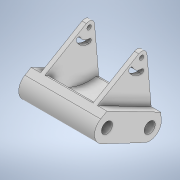
# Autodesk Inventor part: Kauri camera predator mini standoff mount
Saved by Autodesk Inventor 2020 (Build 240168000, 168)
## iProperties
Created: 2022-05-05
Part Number: Kauri camera predator mini standoff mount
Material: Generic
Document SubType Name: Modeling
Designer: Steven
Density: 1 g/cm^3
Appearance: Default
Author: Steven
Autodesk Inventor part; units mm, degrees
ref_plane "YZ Plane" through (0, 0, 0) normal (1, 0, 0) x (0, 1, 0)
ref_plane "XZ Plane" through (0, 0, 0) normal (0, 1, 0) x (-1, 0, 0)
ref_plane "XY Plane" through (0, 0, 0) normal (0, 0, 1) x (1, 0, 0)
sketch "Sketch1" plane through (0, 0, 0) normal (1, 0, 0) x (0, 1, 0)
  circle A0 centre (-9.7574, -19.7073) radius 1.55 construction
  circle A1 centre (0, 0) radius 1.55 construction
  circle A2 centre (-9.7574, -19.7073) radius 2.55
  circle A3 centre (0, 0) radius 2.55
  arc A4 (-12.2239, -24.4871) -> (-4.9776, -22.1738) centre (-9.7574, -19.7073) ccw
  circle A5 centre (0, 0) radius 5.7448
  line L0 (-4.9776, -22.1738) -> (5.1052, -2.6344)
  arc A6 (-4.9776, -22.1738) -> (-12.2239, -24.4871) centre (-9.7574, -19.7073) ccw
  line L1 (-14.5372, -17.2408) -> (-5.1904, 2.4623)
  line L2 (0, 0) -> (0, -35.9972) construction
  dimension "d0" = 5.1
  dimension "d1" = 5.1
  constraints: 7 centre point, 7 point on circle, 6 end point, 4 coincident, 1 tangent, 1 vertical
  measures "d0" diameter of A2
  measures "d1" diameter of A3
extrude "Extrusion1" add sketch "Sketch1" along normal blind 35
sketch "Sketch2" plane through (35, 0, 0) normal (1, 0, 0) x (0, 0, -1)
  circle A0 centre (19.7073, -9.7574) radius 2.55 construction
  line L0 (0, 0) -> (19.7073, -9.7574) construction
  line L1 (9.8536, -4.8787) -> (12.3218, 0.1063) construction
  line L2 (22.1738, -4.9776) -> (2.6344, 5.1052) projected
  line L3 (12.3218, 0.1063) -> (21.4932, 17.8794) construction
  arc A1 (22.837, 15.8783) -> (19.0847, 17.8159) centre (20.3468, 15.6578) ccw
  line L4 (21.4932, 17.8794) -> (29.1107, 13.9486) construction
  line L5 (-2.9001, 4.9591) -> (19.0847, 17.8159)
  arc A2 (2.6344, 5.1052) -> (-2.4623, -5.1904) centre (0, 0) ccw projected
  line L6 (22.837, 15.8783) -> (25.065, -9.283)
  arc A3 (17.2408, -14.5372) -> (22.1738, -4.9776) centre (19.7073, -9.7574) ccw projected
  dimension "d4" = 20
  dimension "d5" = 5
  constraints: 12 end point, 5 tangent, 4 point on circle, 2 perpendicular, 2 point on line, 1 centre point, 1 midpoint
  measures "d4" distance of L1.end L3.end
  measures "d5" diameter of A1
extrude "Extrusion2" add sketch "Sketch2" against normal up to surface (35 mm away)
sketch "Sketch4" plane through (35, 0, 0) normal (1, 0, 0) x (0, 0, -1)
  arc A0 (-2.9001, 4.9591) -> (-2.4623, -5.1904) centre (0, 0) ccw construction
  line L0 (-2.4623, -5.1904) -> (17.2408, -14.5372) construction
  arc A1 (17.2408, -14.5372) -> (25.065, -9.283) centre (19.7073, -9.7574) ccw construction
  line L1 (25.065, -9.283) -> (22.837, 15.8783) construction
  arc A2 (22.837, 15.8783) -> (19.0847, 17.8159) centre (20.3468, 15.6578) ccw construction
  line L2 (19.0847, 17.8159) -> (-2.9001, 4.9591) construction
  circle A3 centre (19.7073, -9.7574) radius 2.55 construction
  circle A4 centre (0, 0) radius 2.55 construction
  circle A5 centre (20.3468, 15.6578) radius 1
  dimension "d8" = 2
  constraints: 1 centre point, 1 coincident
  measures "d8" diameter of A5
extrude "Extrusion3" cut sketch "Sketch4" against normal up to surface (35 mm away)
sketch "Sketch5" plane through (35, 0, 0) normal (1, 0, 0) x (0, 0, -1)
  circle A0 centre (20.3468, 15.6578) radius 1 construction
  arc A1 (-2.9001, 4.9591) -> (-2.4623, -5.1904) centre (0, 0) ccw construction
  line L0 (-2.4623, -5.1904) -> (17.2408, -14.5372) construction
  arc A2 (17.2408, -14.5372) -> (25.065, -9.283) centre (19.7073, -9.7574) ccw construction
  line L1 (25.065, -9.283) -> (22.837, 15.8783) construction
  arc A3 (22.837, 15.8783) -> (19.0847, 17.8159) centre (20.3468, 15.6578) ccw construction
  line L2 (19.0847, 17.8159) -> (-2.9001, 4.9591) construction
  circle A4 centre (19.7073, -9.7574) radius 2.55 construction
  circle A5 centre (0, 0) radius 2.55 construction
  circle A6 centre (19.7073, -9.7574) radius 2.55 construction
  line L3 (0, 0) -> (19.7073, -9.7574) construction
  arc A7 (22.837, 15.8783) -> (19.0847, 17.8159) centre (20.3468, 15.6578) ccw construction
  line L4 (9.8536, -4.8787) -> (20.3468, 15.6578) construction
  circle A8 centre (20.3468, 15.6578) radius 5.5 construction
  circle A9 centre (17.8443, 10.7601) radius 1 construction
  arc A10 (20.3467, 9.1578) -> (20.3468, 11.1578) centre (20.3468, 10.1578) ccw
  arc A11 (16.2684, 13.756) -> (14.4558, 12.9107) centre (15.3621, 13.3334) ccw
  circle A12 centre (20.3468, 15.6578) radius 1 construction
  line L5 (20.3468, 15.6578) -> (20.3468, 10.1578) construction
  line L6 (20.3468, 15.6578) -> (15.3621, 13.3334) construction
  arc A13 (16.2684, 13.756) -> (20.3468, 11.1578) centre (20.3468, 15.6578) ccw
  arc A14 (14.4558, 12.9107) -> (20.3467, 9.1578) centre (20.3469, 15.658) ccw
  arc A15 (19.3509, 10.2487) -> (20.3467, 9.1578) centre (20.3468, 10.1578) ccw construction
  arc A16 (20.3468, 11.1578) -> (19.3509, 10.2487) centre (20.3468, 10.1578) ccw construction
  arc A17 (15.8653, 12.4693) -> (16.2684, 13.756) centre (15.3621, 13.3334) ccw construction
  arc A18 (14.4558, 12.9107) -> (15.8653, 12.4693) centre (15.3621, 13.3334) ccw construction
  dimension "d11" = 11
  dimension "d12" = 2
  dimension "d13" = 2
  dimension "d14" = 2
  dimension "d15" = 65
  constraints: 24 point on circle, 10 centre point, 8 end point, 3 point on line, 1 coincident, 1 midpoint, 1 tangent, 1 vertical
  measures "d11" diameter of A8
  measures "d12" diameter of A9
  measures "d13" diameter of A10
  measures "d14" diameter of A11
  measures "d15" angle of L5 L6
extrude "Extrusion4" cut sketch "Sketch5" against normal up to surface (35 mm away)
ref_plane "Work Plane1" through (0, 19.8068, -22.4892) normal (0, 0.4588093, 0.8885348) x (1, 0, 0)
sketch "Sketch6" plane through (0, 19.8068, -22.4892) normal (0, 0.4588093, 0.8885348) x (1, 0, 0)
  line L0 (35, -25.3672) -> (0, -25.3672) construction
  line L1 (17.5, -24.9952) -> (17.5, 12.8819) construction
  line L2 (17.5, -24.9952) -> (28.6, -24.9952) construction
  line L3 (17.5, -24.9952) -> (6.4, -24.9952) construction
  line L4 (28.6, -24.9952) -> (28.6, -21.9952) construction
  line L5 (6.4, -24.9952) -> (6.4, -21.9952) construction
  line L6 (28.6, -24.9952) -> (28.6, -21.9952) construction
  line L7 (28.6, -21.9952) -> (6.4, -21.9952)
  line L8 (6.4, -21.9952) -> (6.4, 4.5678)
  line L9 (28.6, -21.9952) -> (28.6, 4.5678)
  line L10 (6.4, 4.5678) -> (28.6, 4.5678)
  point P0 (0, -27.9172)
  dimension "d18" = 11.1
  dimension "d19" = 3
  constraints: 20 end point, 5 vertical, 2 perpendicular, 1 horizontal, 1 symmetric about line
  measures "d18" distance of L1.start L2.end
  measures "d19" distance of L2.end L4.end
extrude "Extrusion5" cut sketch "Sketch6" along normal through all both and the other way through all
sketch "Sketch7" plane through (28.6, -6.1337, -24.7861) normal (-1, 0, 0) x (0, 0.4588093, 0.8885348)
  circle A0 centre (13.9427, 17.3257) radius 1 construction
  circle A1 centre (2.8502, -5.55) radius 2.55 construction
  circle A2 centre (24.8375, -5.9221) radius 2.55 construction
  circle A3 centre (2.8502, -5.55) radius 4 construction
  circle A4 centre (24.8375, -5.9221) radius 4 construction
  circle A5 centre (13.9427, 17.3257) radius 21.4232
  dimension "d22" = 8
  dimension "d23" = 8
  constraints: 3 centre point, 3 coincident, 1 tangent
  measures "d22" diameter of A3
  measures "d23" diameter of A4
extrude "Extrusion6" cut sketch "Sketch7" along normal up to surface (22.2 mm away)
sketch "Sketch8" plane through (0, 0, 0) normal (-1, 0, 0) x (0, 0, 1)
  circle A0 centre (-19.7073, -9.7574) radius 2.55 construction
  circle A1 centre (0, 0) radius 2.55 construction
  circle A2 centre (0, 0) radius 5.7448 construction
  circle A3 centre (-19.7073, -9.7574) radius 5.3787 construction
  arc A4 (-23.5937, -5.518) -> (-1.2015, 6.0446) centre (-20.3468, 15.6578) ccw projected
  arc A5 (-20.3467, 9.1578) -> (-14.4558, 12.9107) centre (-20.3469, 15.658) ccw projected
  arc A6 (-20.3468, 11.1578) -> (-20.3467, 9.1578) centre (-20.3468, 10.1578) ccw projected
  arc A7 (-20.3468, 11.1578) -> (-16.2684, 13.756) centre (-20.3468, 15.6578) ccw projected
  arc A8 (-14.4558, 12.9107) -> (-16.2684, 13.756) centre (-15.3621, 13.3334) ccw projected
  circle A9 centre (-20.3468, 15.6578) radius 1 projected
  line L0 (2.9001, 4.9591) -> (-19.0847, 17.8159) projected
  arc A10 (-19.0847, 17.8159) -> (-22.837, 15.8783) centre (-20.3468, 15.6578) ccw projected
  line L1 (-22.837, 15.8783) -> (-25.065, -9.283) projected
  arc A11 (-25.065, -9.283) -> (-17.2408, -14.5372) centre (-19.7073, -9.7574) ccw projected
  line L2 (2.4623, -5.1904) -> (-17.2408, -14.5372) projected
  arc A12 (2.4623, -5.1904) -> (2.9001, 4.9591) centre (0, 0) ccw projected
  circle A13 centre (-19.7073, -9.7574) radius 2.55 projected
  circle A14 centre (0, 0) radius 2.55 projected
  line L3 (-1.2015, 6.0446) -> (-0.009, 6.6603) projected
  line L4 (-24.7861, -6.1337) -> (-23.5937, -5.518) projected
  line L5 (-24.7861, -6.1337) -> (-0.009, 6.6603)
  point P0 (-23.5937, -5.518)
  point P1 (-1.2015, 6.0446)
  constraints: 2 centre point, 2 coincident, 2 end point
extrude "Extrusion7" cut sketch "Sketch8" against normal blind 4.4 contours L4 L1 A10 L0 L3 L5
sketch "Sketch9" plane through (35, 0, 0) normal (1, 0, 0) x (0, 0, -1)
  line L0 (0.009, 6.6603) -> (24.7861, -6.1337) projected
  arc A0 (14.4558, 12.9107) -> (20.3467, 9.1578) centre (20.3469, 15.658) ccw projected
  arc A1 (16.2684, 13.756) -> (14.4558, 12.9107) centre (15.3621, 13.3334) ccw projected
  arc A2 (16.2684, 13.756) -> (20.3468, 11.1578) centre (20.3468, 15.6578) ccw projected
  arc A3 (20.3467, 9.1578) -> (20.3468, 11.1578) centre (20.3468, 10.1578) ccw projected
  circle A4 centre (20.3468, 15.6578) radius 1 projected
  arc A5 (-2.9001, 4.9591) -> (-2.4623, -5.1904) centre (0, 0) ccw projected
  line L1 (-2.4623, -5.1904) -> (17.2408, -14.5372) projected
  arc A6 (17.2408, -14.5372) -> (25.065, -9.283) centre (19.7073, -9.7574) ccw projected
  line L2 (25.065, -9.283) -> (22.837, 15.8783) projected
  arc A7 (22.837, 15.8783) -> (19.0847, 17.8159) centre (20.3468, 15.6578) ccw projected
  line L3 (19.0847, 17.8159) -> (-2.9001, 4.9591) projected
  circle A8 centre (19.7073, -9.7574) radius 2.55 projected
  circle A9 centre (0, 0) radius 2.55 projected
extrude "Extrusion8" cut sketch "Sketch9" against normal blind 4.4 contours L3 A7 L2 L0
body "Solid1"
